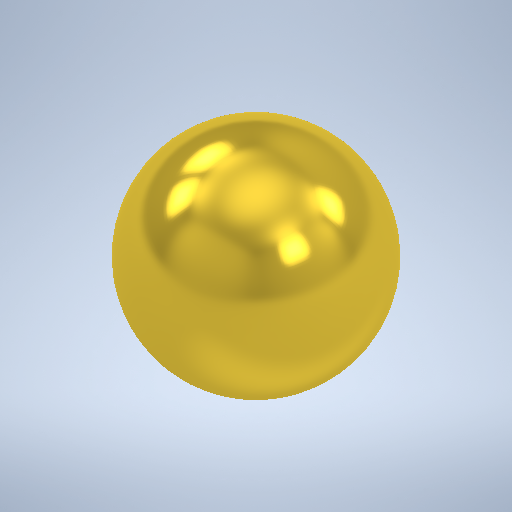
# Autodesk Inventor part: Esfera_0001_001
Saved by Autodesk Inventor 2025.2 (Build 292293000, 293)
## iProperties
Created: 2025-03-26
Part Number: Esfera_0001_001
Material: Ouro
Document SubType Name: Modeling
Designer: lucas
Density: 19.3 g/cm^3
Appearance: Metal quente 2400F
Author: lucas
Autodesk Inventor part; units mm, degrees
ref_plane "YZ Plane" through (0, 0, 0) normal (1, 0, 0) x (0, 1, 0)
ref_plane "XZ Plane" through (0, 0, 0) normal (0, 1, 0) x (-1, 0, 0)
ref_plane "XY Plane" through (0, 0, 0) normal (0, 0, 1) x (1, 0, 0)
sketch "Esboço1" plane through (0, 0, 0) normal (0, 0, 1) x (1, 0, 0)
  circle A0 centre (0, 0) radius 10 construction
  arc A1 (0, -10) -> (0, 10) centre (0, 0) ccw
  line L0 (0, 10) -> (0, 0)
  line L1 (0, 0) -> (0, -10)
  line L2 (0, -14) -> (0, 14) projected
  dimension "d1" = 20
  constraints: 4 end point, 4 point on circle, 2 centre point, 2 vertical alignment, 1 coincident, 1 collinear, 1 concentric, 1 vertical
  measures "d1" diameter of A0
revolve "Revolução1" add sketch "Esboço1" angle 360 about axis through (0, -10, 0) along (0, 1, 0)
